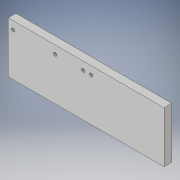
# Autodesk Inventor part: Kermit bumper (medium 3)
Saved by Autodesk Inventor 2018.2 (Build 222227000, 227)
## iProperties
Created: 2018-02-15
Part Number: Kermit bumper (medium 3)
Material: Generic
Document SubType Name: Modeling
Designer: kalra.rohan
Density: 1 g/cm^3
Appearance: Default
Author: kalra.rohan
Autodesk Inventor part; units mm, degrees
ref_plane "YZ Plane" through (0, 0, 0) normal (1, 0, 0) x (0, 1, 0)
ref_plane "XZ Plane" through (0, 0, 0) normal (0, 1, 0) x (-1, 0, 0)
ref_plane "XY Plane" through (0, 0, 0) normal (0, 0, 1) x (1, 0, 0)
sketch "Sketch1" plane through (0, 0, 0) normal (0, 0, 1) x (1, 0, 0)
  line L0 (0, 0) -> (368.3, 0)
  line L1 (368.3, 0) -> (368.3, -120.65)
  line L2 (368.3, -120.65) -> (0, -120.65)
  line L3 (0, -120.65) -> (0, 0)
  circle A0 centre (11.5824, -19.05) radius 3.8672
  circle A1 centre (111.125, -19.05) radius 3.8735
  circle A2 centre (177.3428, -19.05) radius 3.8672
  circle A3 centre (196.1896, -19.05) radius 3.8671
  dimension "d0" = 368.3
  dimension "d1" = 120.65
  dimension "d2" = 7.7343
  dimension "d3" = 101.6
  dimension "d4" = 11.5824
  dimension "d5" = 7.747
  dimension "d6" = 101.6
  dimension "d7" = 99.5426
  dimension "d8" = 7.7343
  dimension "d10" = 66.2178
  dimension "d11" = 7.7343
  dimension "d13" = 18.8468
  dimension "d16" = 101.6
  dimension "d17" = 101.6
  constraints: 8 end point, 4 centre point, 2 parallel, 1 horizontal, 1 perpendicular
  measures "d0" distance between parallel lines of L1 L3
  measures "d1" distance between parallel lines of L0 L2
  measures "d2" diameter of A0
  measures "d3" distance from line of A0.centre L2
  measures "d4" distance from line of A0.centre L3
  measures "d5" diameter of A1
  measures "d6" distance from line of A1.centre L2
  measures "d7" distance of A1.centre A0.centre
  measures "d8" diameter of A2
  measures "d10" distance of A2.centre A1.centre
  measures "d11" diameter of A3
  measures "d13" distance of A3.centre A2.centre
  measures "d16" distance from line of L2 A2.centre
  measures "d17" distance from line of L2 A3.centre
extrude "Extrusion1" add sketch "Sketch1" against normal blind 18.3261
body "Solid1"
